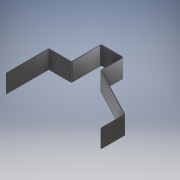
# Autodesk Inventor part: INTERNAL FRAME
Saved by Autodesk Inventor 2018 (Build 220112000, 112)
## iProperties
Created: 2018-10-15
Part Number: INTERNAL FRAME
Material: Acero, carbono
Document SubType Name: Modeling
Designer: Toshiba
Density: 7.85 g/cm^3
Appearance: Mecanizado 02
Author: Toshiba
Autodesk Inventor part; units mm, degrees
ref_plane "YZ Plane" through (0, 0, 0) normal (1, 0, 0) x (0, 1, 0)
ref_plane "XZ Plane" through (0, 0, 0) normal (0, 1, 0) x (-1, 0, 0)
ref_plane "XY Plane" through (0, 0, 0) normal (0, 0, 1) x (1, 0, 0)
sketch "Boceto1" plane through (0, 0, 0) normal (0, 0, 1) x (1, 0, 0)
  line L0 (200, -104) -> (200, -8.6304)
  arc A0 (200, -8.6304) -> (196.784, -3.3155) centre (194, -8.6304) ccw
  line L1 (196.784, -3.3155) -> (-6.784, 103.3155)
  arc A1 (-10, 108.6304) -> (-6.784, 103.3155) centre (-4, 108.6304) ccw
  line L2 (-10, 108.6304) -> (-10, 194)
  arc A2 (-10, 194) -> (-16, 200) centre (-16, 194) ccw
  line L3 (-16, 200) -> (-99, 200)
  arc A3 (-99, 200) -> (-105, 194) centre (-99, 194) ccw
  line L4 (-105, 194) -> (-105, 77)
  arc A4 (-107, 75) -> (-105, 77) centre (-107, 77) ccw
  line L5 (-107, 75) -> (-173, 75)
  arc A5 (-175, 123) -> (-177, 125) centre (-177, 123) ccw
  line L6 (-200, 75) -> (-200, -104)
  line L7 (-173, 75) -> (-200, 75)
  line L8 (-198, 73) -> (-173, 73)
  line L9 (-173, 73) -> (-107, 73)
  arc A6 (-107, 73) -> (-103, 77) centre (-107, 77) ccw
  line L10 (-103, 77) -> (-103, 194)
  arc A7 (-99, 198) -> (-103, 194) centre (-99, 194) ccw
  line L11 (-99, 198) -> (-16, 198)
  arc A8 (-12, 194) -> (-16, 198) centre (-16, 194) ccw
  line L12 (-12, 194) -> (-12, 108.6304)
  arc A9 (-12, 108.6304) -> (-7.7121, 101.5438) centre (-4, 108.6304) ccw
  line L13 (-7.7121, 101.5438) -> (195.856, -5.0871)
  arc A10 (198, -8.6304) -> (195.856, -5.0871) centre (194, -8.6304) ccw
  line L14 (198, -8.6304) -> (198, -104)
  line L15 (-198, 73) -> (-198, -104)
  line L16 (-200, -104) -> (-198, -104)
  line L17 (198, -104) -> (200, -104)
  point P0 (0, 0)
  dimension "d3" = 2
  dimension "d4" = 2
  constraints: 37 end point, 22 point on circle, 11 centre point, 2 point on line, 1 collinear, 1 horizontal, 1 parallel, 1 perpendicular, 11 other
  measures "d3" distance between parallel lines of L4 L10
  measures "d4" distance between parallel lines of L6 L15
extrude "Extrusión1" add sketch "Boceto1" along normal mid plane 75
